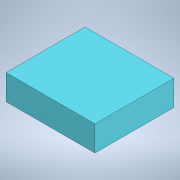
# Autodesk Inventor part: caseUpperPortionV02
Saved by Autodesk Inventor 2022.2 (Build 262287000, 287)
## iProperties
Created: 2021-08-20
Part Number: caseUpperPortionV02
Material: PC/ABS Plastic
Document SubType Name: Modeling
Designer: robst
Density: 0.357273 g/cm^3
Appearance: Cadet Blue
Author: robst
Autodesk Inventor part; units mm, degrees
ref_plane "YZ Plane" through (0, 0, 0) normal (1, 0, 0) x (0, 1, 0)
ref_plane "XZ Plane" through (0, 0, 0) normal (0, 1, 0) x (-1, 0, 0)
ref_plane "XY Plane" through (0, 0, 0) normal (0, 0, 1) x (1, 0, 0)
sketch "Sketch33" plane through (0, 0, 0) normal (0, 1, 0) x (-1, 0, 0)
  line L0 (68.5, 60.85) -> (-68.5, 60.85)
  line L1 (-68.5, 60.85) -> (-68.5, -60.85)
  line L2 (-68.5, -60.85) -> (68.5, -60.85)
  line L3 (68.5, -60.85) -> (68.5, 60.85)
  line L4 (68.5, 60.85) -> (-68.5, -60.85) construction
  line L5 (-68.5, 60.85) -> (68.5, -60.85) construction
  line L6 (58.5, 50.85) -> (-58.5, 50.85)
  line L7 (-58.5, 50.85) -> (-58.5, -50.85)
  line L8 (-58.5, -50.85) -> (58.5, -50.85)
  line L9 (58.5, -50.85) -> (58.5, 50.85)
  line L10 (58.5, 50.85) -> (-58.5, -50.85) construction
  line L11 (-58.5, 50.85) -> (58.5, -50.85) construction
  point P0 (0, 0)
  dimension "d178" = 121.7
  dimension "d179" = 137
  dimension "d180" = 10
  dimension "d181" = 10
  constraints: 24 end point, 4 midpoint, 4 parallel, 2 horizontal, 2 perpendicular
  measures "d178" distance of L2.end L0.start
  measures "d179" distance of L1.end L2.end
  measures "d180" distance between parallel lines of L8 L2
  measures "d181" distance between parallel lines of L3 L9
extrude "Extrusion26" add sketch "Sketch33" along normal blind 8 contours L3 L2 L1 L0 | L9 L8 L7 L6
extrude "Extrusion27" add sketch "Sketch33" against normal blind 31
equation "\"caseWidth\" = 137"
equation "\"thickenDistance\" = 1"
equation "\"caseDepth\" = 31"
equation "\"caseLength\" = 121.7"
equation "\"d95\" = lensDiameter"
equation "\"topWallThickness\" = 8"
equation "\"lensDiameter\" = 15"
body "Solid2"
